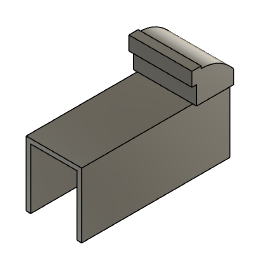
Slider (Autodesk Fusion 360 design; units mm, degrees)
Autodesk Fusion 360 part; units mm, degrees
sketch "Sketch2" plane through (0, 0, 0) normal (0, 1, 0) x (1, 0, 0)
  line L0 (38.1, -44.45) -> (-38.1, -44.45)
  line L1 (-38.1, -44.45) -> (-38.1, 44.45)
  line L2 (-38.1, 44.45) -> (38.1, 44.45)
  line L3 (38.1, 44.45) -> (38.1, -44.45)
  line L4 (38.1, -44.45) -> (-38.1, 44.45) construction
  line L5 (-38.1, -44.45) -> (38.1, 44.45) construction
  dimension "d3" = 76.2
  dimension "d4" = 88.9
  constraint horizontal L0
  constraint perpendicular L0 L1
  constraint parallel L0 L2
  constraint parallel L1 L3
  constraint coincident L4 origin
  constraint coincident L5 origin
  measures "d3" distance of L1.end L2.end
  measures "d4" distance of L0.end L1.end
extrude "Extrude1" add sketch "Sketch2" along normal blind 203.2
sketch "Sketch3" plane through (0, 0, 0) normal (0, -1, 0) x (1, 0, 0)
  line L0 (-38.1, -44.45) -> (38.1, -44.45)
  line L1 (38.1, -44.45) -> (38.1, 44.45)
  line L2 (38.1, 44.45) -> (-38.1, 44.45)
  line L3 (-38.1, 44.45) -> (-38.1, -44.45)
  line L4 (-31.75, -44.45) -> (31.75, -44.45)
  line L5 (31.75, -44.45) -> (31.75, 38.1)
  line L6 (31.75, 38.1) -> (-31.75, 38.1)
  line L7 (-31.75, 38.1) -> (-31.75, -44.45)
  dimension "d7" = 63.5
  dimension "d8" = 6.35
  dimension "d9" = 6.35
  constraint horizontal L4
  constraint vertical L5
  constraint horizontal L6
  constraint vertical L7
  constraint collinear L0 L4
  measures "d7" distance of L4.start L4.end
  measures "d8" distance of L1 L5
  measures "d9" distance of L2 L6
extrude "Extrude2" cut sketch "Sketch3" against normal blind 190.5 contours L0 L4 L5 L6 L7
sketch "Sketch4" plane through (38.1, 0, 0) normal (1, 0, 0) x (0, 1, 0)
  line L0 (0, 44.45) -> (0, -44.45)
  line L1 (0, -44.45) -> (203.2, -44.45)
  line L2 (203.2, -44.45) -> (203.2, 44.45)
  line L3 (203.2, 44.45) -> (0, 44.45)
  line L4 (152.4, 63.4925) -> (203.2, 63.4925)
  line L5 (152.4, 63.4925) -> (152.4, 69.8425)
  line L6 (152.4, 69.8425) -> (158.75, 69.8425)
  line L7 (158.75, 69.8425) -> (158.75, 85.7937)
  line L8 (152.4, 63.4925) -> (152.4, 44.45)
  line L9 (203.2, 63.4925) -> (203.2, 44.45)
  spline S0 degree 5 poles (203.2, 63.4925) (202.0453, 64.8323) (199.6635, 67.4597) (195.8735, 71.2447) (190.3554, 75.9576) (182.304, 81.0202) (174.3584, 83.9897) (167.1278, 85.3037) (161.6519, 85.7089) (158.75, 85.7937) knots 0 0 0 0 0 0 0.2 0.4 0.6 0.8 1 1 1 1 1 1
  line L10 (165.8196, 85.5871) -> (151.6804, 86.0004)
  dimension "d12" = 50.8
  dimension "d13" = 6.35
  dimension "d14" = 15.9512
  dimension "d27" = 19.0426
  dimension "d28" = 6.35
  constraint perpendicular L0 L4
  constraint perpendicular L4 L5
  constraint perpendicular L5 L6
  constraint perpendicular L6 L7
  constraint coincident L3 L8.end
  constraint perpendicular L3 L8
  constraint coincident L3 L2.end
  constraint perpendicular L3 L9
  constraint coincident L2.end L3.start
  constraint midpoint L7.end L10
  measures "d12" distance of L4.start L4.end
  measures "d13" distance of L5.end L6.end
  measures "d14" distance of L6.end L7.end
  measures "d27" distance of L4.start L8.end
  measures "d28" distance of L4.start L5.end
extrude "Extrude3" add sketch "Sketch4" along normal blind 5.08 and the other way blind 81.28 contours L3 L4 L8 L9 | L4 L5 L6 L7 S0
sketch "Sketch5" plane through (0, 158.75, 0) normal (0, -1, 0) x (1, 0, 0)
  line L0 (43.18, 69.8425) -> (43.18, 85.7937)
  line L1 (-43.18, 69.8425) -> (43.18, 69.8425)
  line L2 (-43.18, 85.7937) -> (-43.18, 69.8425)
  line L3 (43.18, 69.8425) -> (-43.18, 69.8425)
  line L4 (-43.18, 69.8425) -> (43.18, 69.8425)
  line L5 (43.18, 69.8425) -> (43.18, 88.8925)
  line L6 (43.18, 88.8925) -> (-43.18, 88.8925)
  line L7 (-43.18, 88.8925) -> (-43.18, 69.8425)
  line L8 (43.18, 85.7937) -> (-43.18, 85.7937)
  dimension "d26" = 19.05
  constraint horizontal L3
  constraint coincident L0.start L1.end
  constraint horizontal L4
  constraint vertical L5
  constraint horizontal L6
  constraint vertical L7
  constraint collinear L0 L5
  constraint collinear L2 L7
  measures "d26" distance of L1.start L6.end
extrude "Extrude4" add sketch "Sketch5" along normal blind 12.7
sketch "Sketch6" plane through (0, 203.2, 0) normal (0, 1, 0) x (-1, 0, 0)
  line L0 (-38.1, -44.45) -> (38.1, -44.45)
  line L1 (38.1, -44.45) -> (38.1, 44.45)
  line L2 (38.1, 44.45) -> (43.18, 44.45)
  line L3 (-43.18, 63.4925) -> (-43.18, 44.45)
  line L4 (43.18, 44.45) -> (43.18, 63.4925)
  line L5 (-38.1, 44.45) -> (-38.1, -44.45)
  circle A0 centre (-0.0873, -17.907) radius 12.7
  line L6 (-0.0873, 10.16) -> (-0.0873, -53.34) construction
  line L7 (43.18, 63.4925) -> (-43.18, 63.4925)
  line L8 (-43.18, 44.45) -> (-38.1, 44.45)
  dimension "d23" = 25.4
  dimension "d25" = 26.543
  constraint perpendicular L0 L6
  constraint coincident A0.centre L6
  measures "d23" diameter of A0
  measures "d25" distance of L0 A0.centre
extrude "Extrude5" cut sketch "Sketch6" against normal through all contours A0
